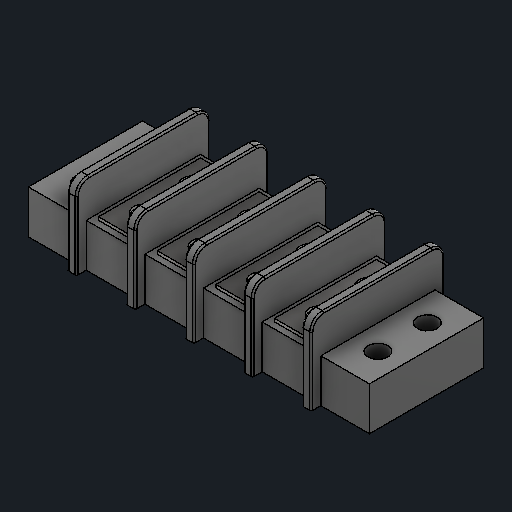
# Autodesk Inventor part: Terminal Block
Saved by Autodesk Inventor 2026.2 (Build 302298000, 298)
## iProperties
Created: 2026-08-15
Part Number: Terminal Block
Material: PC/ABS Plastic
Document SubType Name: Modeling
Designer: JoshuaEah
Density: 1.1 g/cm^3
Appearance: Smooth - Black
Author: JoshuaEah
Autodesk Inventor part; units mm, degrees
ref_plane "YZ Plane" through (0, 0, 0) normal (1, 0, 0) x (0, 1, 0)
ref_plane "XZ Plane" through (0, 0, 0) normal (0, 1, 0) x (-1, 0, 0)
ref_plane "XY Plane" through (0, 0, 0) normal (0, 0, 1) x (1, 0, 0)
sketch "Sketch1" plane through (0, 0, 0) normal (0, 1, 0) x (-1, 0, 0)
  line L0 (0, 0) -> (-55.25, 0)
  line L1 (-55.25, 0) -> (-55.25, -18.5)
  line L2 (-55.25, -18.5) -> (0, -18.5)
  line L3 (0, -18.5) -> (0, 0)
  line L4 (-27.625, -18.5) -> (-27.625, 0)
  line L5 (-26.875, -20.05) -> (-28.375, -20.05)
  line L6 (-28.375, -20.05) -> (-28.375, 1.55)
  line L7 (-28.375, 1.55) -> (-26.875, 1.55)
  line L8 (-26.875, 1.55) -> (-26.875, -20.05)
  line L9 (-17.375, 1.55) -> (-17.375, -20.05)
  line L10 (-17.375, -20.05) -> (-18.875, -20.05)
  line L11 (-18.875, -20.05) -> (-18.875, 1.55)
  line L12 (-18.875, 1.55) -> (-17.375, 1.55)
  line L13 (-36.375, 1.55) -> (-36.375, -20.05)
  line L14 (-36.375, -20.05) -> (-37.875, -20.05)
  line L15 (-37.875, -20.05) -> (-37.875, 1.55)
  line L16 (-37.875, 1.55) -> (-36.375, 1.55)
  line L17 (-7.875, 1.55) -> (-7.875, -20.05)
  line L18 (-7.875, -20.05) -> (-9.375, -20.05)
  line L19 (-9.375, -20.05) -> (-9.375, 1.55)
  line L20 (-9.375, 1.55) -> (-7.875, 1.55)
  line L21 (-45.875, 1.55) -> (-45.875, -20.05)
  line L22 (-45.875, -20.05) -> (-47.375, -20.05)
  line L23 (-47.375, -20.05) -> (-47.375, 1.55)
  line L24 (-47.375, 1.55) -> (-45.875, 1.55)
  line L25 (0, -9.25) -> (-55.25, -9.25)
  line L26 (-19.875, -17.5) -> (-25.875, -17.5)
  line L27 (-25.875, -17.5) -> (-25.875, -1)
  line L28 (-25.875, -1) -> (-19.875, -1)
  line L29 (-19.875, -1) -> (-19.875, -17.5)
  point P0 (-27.625, -9.25)
  point P1 (-28.375, -9.25)
  point P2 (-27.625, -20.05)
  point P3 (-18.125, -20.05)
  point P4 (-18.875, -9.25)
  point P5 (-37.125, -20.05)
  point P6 (-37.875, -9.25)
  point P7 (-8.625, -20.05)
  point P8 (-9.375, -9.25)
  point P9 (-46.625, -20.05)
  point P10 (-47.375, -9.25)
  point P11 (-3.875, -13.25)
  point P12 (-51.375, -13.25)
  point P13 (-51.375, -5.25)
  point P14 (-3.875, -5.25)
  point P15 (-22.875, -13.25)
  point P16 (-22.875, -5.25)
  point P17 (-22.875, -17.5)
  dimension "d0" = 55.25
  dimension "d1" = 18.5
  dimension "d4" = 21.6
  dimension "d5" = 1.5
  dimension "d8" = 9.5
  dimension "d13" = 47.5
  dimension "d14" = 8
  dimension "d15" = 8
  dimension "d16" = 47.5
  dimension "d32" = 1
  dimension "d33" = 1
  dimension "d34" = 1
  dimension "d35" = 1
  constraints: 60 end point, 8 midpoint, 6 parallel, 5 horizontal alignment, 5 vertical alignment, 4 horizontal, 3 perpendicular, 1 coincident, 40 other
  measures "d0" distance of L2.end L1.end
  measures "d1" distance of L1.end L0.end
  measures "d4" distance of L5.end L6.end
  measures "d5" distance of L5.start L5.end
  measures "d8" distance of L7.end L9.start
  measures "d13" distance of point (-51.375, -13.25) point (-3.875, -13.25)
  measures "d14" distance of point (-3.875, -5.25) point (-3.875, -13.25)
  measures "d15" diameter of point (-3.875, -13.25) L25
  measures "d16" diameter of point (-3.875, -13.25) L4
  measures "d32" distance between parallel lines of L11 L29
  measures "d33" distance between parallel lines of L8 L27
  measures "d34" distance between parallel lines of L2 L26
  measures "d35" distance between parallel lines of L0 L28
extrude "Extrusion1" add sketch "Sketch1" against normal blind 7 contours L3 L25 L17 L0 | L17 L25 L19 L0 | L3 L2 L17 L25 | L19 L25 L9 L0 | L17 L2 L19 L25 | L9 L25 L11 L0 | L19 L2 L9 L25 | L11 L25 L29 L28 L27 L8 L0 | L9 L2 L11 L25 | L8 L25 L4 L0 | L11 L2 L8 L25 L27 L26 L29 | L4 L25 L6 L0 | L8 L2 L4 L25 | L29 L26 L27 L25 | L25 L27 L28 L29 | L6 L25 L13 L0 | L4 L2 L6 L25 | L13 L25 L15 L0 | L6 L2 L13 L25 | L15 L25 L21 L0 | L13 L2 L15 L25 | L21 L25 L23 L0 | L15 L2 L21 L25 | L23 L25 L1 L0 | L21 L2 L23 L25 | L23 L2 L1 L25
extrude "Extrusion2" add sketch "Sketch1" along normal blind 6 and the other way blind 7 contours L17 L25 L19 L0 | L0 L19 L20 L17 | L17 L2 L19 L25 | L9 L25 L11 L0 | L0 L11 L12 L9 | L17 L18 L19 L2 | L9 L2 L11 L25 | L8 L25 L4 L0 | L0 L6 L7 L8 | L9 L10 L11 L2 | L4 L25 L6 L0 | L8 L2 L4 L25 | L4 L2 L6 L25 | L8 L5 L6 L2 | L13 L25 L15 L0 | L0 L15 L16 L13 | L13 L2 L15 L25 | L21 L25 L23 L0 | L0 L23 L24 L21 | L13 L14 L15 L2 | L21 L2 L23 L25 | L21 L22 L23 L2
fillet "Fillet1" radius 2 10 edges at (46.625, 6, 1.55) (46.625, 6, -20.05) (37.125, 6, -20.05) (37.125, 6, 1.55) (27.625, 6, 1.55) (27.625, 6, -20.05) (18.125, 6, -20.05) (18.125, 6, 1.55) (8.625, 6, -20.05) (8.625, 6, 1.55)
fillet "Fillet2" radius 0.25 50 edges at (47.375, 5.4142, -19.4642) (47.375, -1.5, -20.05) (47.375, 5.4142, 0.9642) (47.375, -1.5, 1.55) (47.375, 6, -9.25) (45.875, 5.4142, 0.9642) (45.875, -1.5, 1.55) (45.875, 5.4142, -19.4642) (45.875, -1.5, -20.05) (45.875, 6, -9.25) (37.875, 5.4142, -19.4642) (37.875, -1.5, -20.05) (37.875, 5.4142, 0.9642) (37.875, -1.5, 1.55) (37.875, 6, -9.25) (36.375, 5.4142, 0.9642) (36.375, -1.5, 1.55) (36.375, 5.4142, -19.4642) (36.375, -1.5, -20.05) (36.375, 6, -9.25) (28.375, 5.4142, -19.4642) (28.375, -1.5, -20.05) (28.375, 5.4142, 0.9642) (28.375, -1.5, 1.55) (28.375, 6, -9.25) (26.875, 5.4142, 0.9642) (26.875, -1.5, 1.55) (26.875, 5.4142, -19.4642) (26.875, -1.5, -20.05) (26.875, 6, -9.25) (18.875, 5.4142, -19.4642) (18.875, -1.5, -20.05) (18.875, 5.4142, 0.9642) (18.875, -1.5, 1.55) (18.875, 6, -9.25) (17.375, 5.4142, 0.9642) (17.375, -1.5, 1.55) (17.375, 5.4142, -19.4642) (17.375, -1.5, -20.05) (17.375, 6, -9.25) (9.375, 5.4142, -19.4642) (9.375, -1.5, -20.05) (9.375, 5.4142, 0.9642) (9.375, -1.5, 1.55) (9.375, 6, -9.25) (7.875, 5.4142, 0.9642) (7.875, -1.5, 1.55) (7.875, 5.4142, -19.4642) (7.875, -1.5, -20.05) (7.875, 6, -9.25)
hole "Hole1" at (3.875, 0, -13.25) at (51.375, 0, -13.25) at (51.375, 0, -5.25) at (3.875, 0, -5.25) direction (0, -1, 0) diameter 3.2004 end through all clearance for "Socket Head Cap Screw" size "M3" standard "Ansi Metric M Profile"
extrude "Extrusion3" add sketch "Sketch1" along normal blind 0.5 separate body contours L29 L26 L27 L25 | L25 L27 L28 L29
hole "Hole2" at (22.875, 0, -13.25) at (22.875, 0, -5.25) direction (0, 1, 0) diameter 3.2004 depth 0.5 bodies 2 clearance for "Socket Head Cap Screw" size "M3" standard "Ansi Metric M Profile"
pattern_linear "Rectangular Pattern1" count 4 spacing 9.5 along (1, 0, 0) of "Extrusion3", "Hole2" first direction both ways yes bodies 2
equation "\"d15\" = d14"
equation "\"d16\" = d13"
body "Solid1"
body "Solid2"
